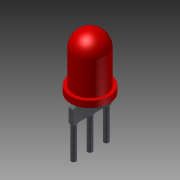
# Autodesk Inventor part: LED
Saved by Autodesk Inventor 2012 (Build 160160000, 160)
## iProperties
Created: 2013-12-16
Part Number: LED
Material: Default
Document SubType Name: Modeling
Designer: joe_000
Density: 1 g/cm^3
Author: joe_000
Autodesk Inventor part; units mm, degrees
ref_plane "YZ Plane" through (0, 0, 0) normal (1, 0, 0) x (0, 1, 0)
ref_plane "XZ Plane" through (0, 0, 0) normal (0, 1, 0) x (-1, 0, 0)
ref_plane "XY Plane" through (0, 0, 0) normal (0, 0, 1) x (1, 0, 0)
sketch "Sketch1" plane through (0, 0, 0) normal (0, 0, 1) x (1, 0, 0)
  circle A0 centre (0, 0) radius 2.5
  dimension "d0" = 5
  constraints: 1 centre point, 1 coincident
  measures "d0" diameter of A0
extrude "Extrusion1" add sketch "Sketch1" along normal blind 5.1
sketch "Sketch2" plane through (0, 0, 0) normal (0, 0, -1) x (-1, 0, 0)
  circle A0 centre (0, 0) radius 2.5
  arc A1 (-0.031716, 2.999832) -> (2.751366, 1.195821) centre (0, 0) ccw
  line L0 (-0.031716, 2.999832) -> (2.751366, 1.195821)
  dimension "d3" = 6
  constraints: 2 end point, 2 point on circle, 1 centre point, 1 coincident, 1 tangent
  measures "d3" diameter of A1
extrude "Extrusion2" add sketch "Sketch2" along normal blind 1 contours A0 | L0 A1
sketch "Sketch4" plane through (0, 0, 0) normal (0, 1, 0) x (-1, 0, 0)
  line L0 (0, 0) -> (0, 10.583317)
  arc A0 (0, 7.5) -> (-2.5, 5) centre (0, 5) ccw
  line L1 (-2.5, 5) -> (0, 5)
  dimension "d11" = 2.5
  dimension "d12" = 5
  constraints: 4 end point, 2 point on circle, 2 point on line, 1 centre point, 1 horizontal, 1 vertical
  measures "d11" radius of A0
  measures "d12" distance of L0.start L1.end
revolve "Revolution1" add sketch "Sketch4" angle 360 about axis through (0, 0, 0) along (0, 0, 1)
sketch "Sketch5" plane through (0, 0, 0) normal (1, 0, 0) x (0, 1, 0)
  line L0 (-2.165084, -1) -> (-2.915084, -1.75)
  line L1 (-2.915084, -1.75) -> (-2.915084, -3.85)
  line L2 (-2.915084, -3.85) -> (-2.165084, -3.85)
  line L3 (-2.165084, -3.85) -> (-2.165084, -3.75)
  line L4 (-2.165084, -3.75) -> (-0.375084, -3.75)
  line L5 (-0.375084, -3.75) -> (-0.375084, -3.85)
  line L6 (-0.375084, -3.85) -> (0.374916, -3.85)
  line L7 (0.374916, -3.85) -> (0.374916, -3.75)
  line L8 (0.374916, -3.75) -> (2.164916, -3.75)
  line L9 (2.164916, -3.75) -> (2.164916, -3.85)
  line L10 (2.164916, -3.85) -> (2.914916, -3.85)
  line L11 (2.914916, -3.85) -> (2.914916, -1.75)
  line L12 (2.914916, -1.75) -> (2.334916, -1)
  line L13 (2.334916, -1) -> (-2.165084, -1)
  line L14 (2.999832, -1) -> (-3, -1)
  line L15 (-0.000084, -1) -> (-0.000084, -3.532862)
  point P0 (0, 0)
  point P1 (1.195821, -1)
  dimension "d14" = 0.75
  dimension "d15" = 0.75
  dimension "d16" = 0.75
  dimension "d17" = 2.54
  dimension "d18" = 2.54
  dimension "d19" = 2.75
  dimension "d20" = 4.5
  dimension "d21" = 0.75
  dimension "d22" = 0.75
  dimension "d23" = 0.1
  dimension "d24" = 0
  dimension "d25" = 0.375
  constraints: 30 end point, 12 perpendicular, 3 collinear, 1 horizontal alignment, 1 midpoint, 1 vertical
  measures "d14" distance of L5.end L6.end
  measures "d15" distance of L1.end L2.end
  measures "d16" distance of L9.end L10.end
  measures "d17" distance of L5.end L1.end
  measures "d18" distance of L9.end L5.end
  measures "d19" distance between parallel lines of L13 L4
  measures "d20" distance of L12.end L0.start
  measures "d21" distance from line of L0.start L1
  measures "d22" distance from line of L11.end L13
  measures "d23" distance of L8.end L9.end
  measures "d24" distance between parallel lines of L14 L13
  measures "d25" distance between parallel lines of L7 L15
extrude "Extrusion3" add sketch "Sketch5" along normal mid plane 0.75
sketch "Sketch6" plane through (0.375, -0.375084, -3.85) normal (0, 0, -1) x (-1, 0, 0)
  line L0 (0, 0) -> (0.75, 0.75)
  line L1 (0.75, 0) -> (0, 0.75)
  circle A0 centre (0.375, 0.375084) radius 0.375
  point P0 (0.375, 0.375084)
  constraints: 4 end point, 1 centre point, 1 coincident, 1 perpendicular
sketch "Sketch7" plane through (0.375, 2.164916, -3.85) normal (0, 0, -1) x (-1, 0, 0)
  line L0 (0, 0.75) -> (0.75, 0)
  line L1 (0.75, 0.75) -> (0, 0)
  circle A0 centre (0.375, 0.375) radius 0.375
  point P0 (0.375, -2.164916)
  constraints: 4 end point, 1 centre point, 1 midpoint, 1 perpendicular
sketch "Sketch8" plane through (0.375, -2.915084, -3.85) normal (0, 0, -1) x (-1, 0, 0)
  line L0 (0, 0.75) -> (0.75, 0)
  line L1 (0.75, 0.75) -> (0, 0)
  circle A0 centre (0.375, 0.375) radius 0.375
  point P0 (0.375, 2.915084)
  constraints: 4 end point, 1 centre point, 1 midpoint, 1 perpendicular
extrude "Extrusion4" add sketch "Sketch8" along normal blind 5
extrude "Extrusion5" add sketch "Sketch6" along normal blind 5
extrude "Extrusion6" add sketch "Sketch7" along normal blind 5
body "Solid1"
